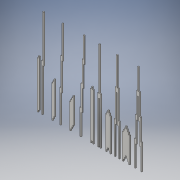
# Autodesk Inventor part: lift drawing
Saved by Autodesk Inventor 2016 SP2 (Build 200236200, 236)
## iProperties
Created: 2018-01-12
Part Number: lift drawing
Material: Generic
Document SubType Name: Modeling
Designer: CAD
Density: 1 g/cm^3
Appearance: Default
Author: CAD
Autodesk Inventor part; units mm, degrees
ref_plane "YZ Plane" through (0, 0, 0) normal (1, 0, 0) x (0, 1, 0)
ref_plane "XZ Plane" through (0, 0, 0) normal (0, 1, 0) x (-1, 0, 0)
ref_plane "XY Plane" through (0, 0, 0) normal (0, 0, 1) x (1, 0, 0)
sketch "Sketch1" plane through (0, 0, 0) normal (0, 0, 1) x (1, 0, 0)
  line L0 (0, 0) -> (2540, 0)
  line L1 (0, 0) -> (0, 1117.6)
  line L2 (0, 1117.6) -> (25.4, 1117.6)
  line L3 (25.4, 49.2125) -> (25.4, 1166.8125)
  line L4 (50.8, 49.2125) -> (50.8, 1166.8125)
  line L5 (25.4, 1166.8125) -> (50.8, 1166.8125)
  line L6 (50.8, 49.2125) -> (25.4, 49.2125)
  line L7 (25.4, 1117.6) -> (25.4, 0)
  line L8 (103.983, 0) -> (103.983, 1117.6)
  line L9 (103.983, 1117.6) -> (129.383, 1117.6)
  line L10 (129.383, 1117.6) -> (129.383, 0)
  line L11 (129.383, 1016) -> (129.383, 2133.6)
  line L12 (129.383, 2133.6) -> (154.783, 2133.6)
  line L13 (154.783, 2133.6) -> (154.783, 1016)
  line L14 (154.783, 1016) -> (129.383, 1016)
  line L15 (346.5563, 0) -> (346.5563, 774.7)
  line L16 (371.9563, 0) -> (371.9563, 774.7)
  line L17 (346.5563, 774.7) -> (371.9563, 774.7)
  line L18 (346.5563, 0) -> (371.9563, 0)
  line L19 (371.9563, 49.2125) -> (371.9563, 823.9125)
  line L20 (397.3563, 49.2125) -> (397.3563, 823.9125)
  line L21 (371.9563, 823.9125) -> (397.3563, 823.9125)
  line L22 (397.3563, 49.2125) -> (371.9563, 49.2125)
  line L23 (397.3563, 98.425) -> (397.3563, 873.125)
  line L24 (422.7563, 98.425) -> (422.7563, 873.125)
  line L25 (422.7563, 98.425) -> (397.3563, 98.425)
  line L26 (397.3563, 873.125) -> (422.7563, 873.125)
  line L27 (536.8328, 0) -> (536.8328, 774.7)
  line L28 (562.2328, 0) -> (562.2328, 774.7)
  line L29 (536.8328, 774.7) -> (562.2328, 774.7)
  line L30 (536.8328, 0) -> (562.2328, 0)
  line L31 (562.2328, 673.1) -> (562.2328, 1447.8)
  line L32 (587.6328, 673.1) -> (587.6328, 1447.8)
  line L33 (587.6328, 673.1) -> (562.2328, 673.1)
  line L34 (587.6328, 1447.8) -> (562.2328, 1447.8)
  line L35 (587.6328, 1346.2) -> (587.6328, 2120.9)
  line L36 (613.0328, 1346.2) -> (613.0328, 2120.9)
  line L37 (613.0328, 1346.2) -> (587.6328, 1346.2)
  line L38 (587.6328, 2120.9) -> (613.0328, 2120.9)
  line L39 (773.9353, 0) -> (773.9353, 609.6)
  line L40 (799.3353, 0) -> (799.3353, 609.6)
  line L41 (773.9353, 609.6) -> (799.3353, 609.6)
  line L42 (799.3353, 0) -> (773.9353, 0)
  line L43 (799.3353, 49.2125) -> (799.3353, 658.8125)
  line L44 (824.7353, 49.2125) -> (824.7353, 658.8125)
  line L45 (824.7353, 658.8125) -> (799.3353, 658.8125)
  line L46 (824.7353, 49.2125) -> (799.3353, 49.2125)
  line L47 (824.7353, 98.425) -> (824.7353, 708.025)
  line L48 (850.1353, 98.425) -> (850.1353, 708.025)
  line L49 (824.7353, 708.025) -> (850.1353, 708.025)
  line L50 (850.1353, 98.425) -> (824.7353, 98.425)
  line L51 (850.1353, 147.6375) -> (850.1353, 757.2375)
  line L52 (875.5353, 147.6375) -> (875.5353, 757.2375)
  line L53 (850.1353, 757.2375) -> (875.5353, 757.2375)
  line L54 (875.5353, 147.6375) -> (850.1353, 147.6375)
  line L55 (1020.3359, 0) -> (1020.3359, 609.6)
  line L56 (1045.7359, 0) -> (1045.7359, 609.6)
  line L57 (1045.7359, 609.6) -> (1020.3359, 609.6)
  line L58 (1020.3359, 0) -> (1045.7359, 0)
  line L59 (1045.7359, 508) -> (1045.7359, 1117.6)
  line L60 (1071.1359, 508) -> (1071.1359, 1117.6)
  line L61 (1071.1359, 508) -> (1045.7359, 508)
  line L62 (1071.1359, 1117.6) -> (1045.7359, 1117.6)
  line L63 (1071.1359, 1016) -> (1071.1359, 1625.6)
  line L64 (1096.5359, 1016) -> (1096.5359, 1625.6)
  line L65 (1096.5359, 1625.6) -> (1071.1359, 1625.6)
  line L66 (1096.5359, 1016) -> (1071.1359, 1016)
  line L67 (1096.5359, 2133.6) -> (1096.5359, 1524)
  line L68 (1121.9359, 2133.6) -> (1121.9359, 1524)
  line L69 (1096.5359, 2133.6) -> (1121.9359, 2133.6)
  line L70 (1121.9359, 1524) -> (1096.5359, 1524)
  line L71 (1631.5096, 0) -> (1631.5096, 774.7)
  line L72 (1656.9096, 0) -> (1656.9096, 774.7)
  line L73 (1631.5096, 774.7) -> (1656.9096, 774.7)
  line L74 (1631.5096, 0) -> (1656.9096, 0)
  line L75 (1656.9096, 49.2125) -> (1656.9096, 823.9125)
  line L76 (1682.3096, 49.2125) -> (1682.3096, 823.9125)
  line L77 (1656.9096, 823.9125) -> (1682.3096, 823.9125)
  line L78 (1682.3096, 49.2125) -> (1656.9096, 49.2125)
  line L79 (1682.3096, 98.425) -> (1682.3096, 873.125)
  line L80 (1707.7096, 98.425) -> (1707.7096, 873.125)
  line L81 (1707.7096, 98.425) -> (1682.3096, 98.425)
  line L82 (1682.3096, 873.125) -> (1707.7096, 873.125)
  line L83 (1733.1096, 0) -> (1733.1096, 774.7)
  line L84 (1758.5096, 0) -> (1758.5096, 774.7)
  line L85 (1733.1096, 774.7) -> (1758.5096, 774.7)
  line L86 (1733.1096, 0) -> (1758.5096, 0)
  line L87 (1733.1096, 823.9125) -> (1707.7096, 823.9125)
  line L88 (1733.1096, 49.2125) -> (1733.1096, 823.9125)
  line L89 (1707.7096, 49.2125) -> (1707.7096, 823.9125)
  line L90 (1707.7096, 49.2125) -> (1733.1096, 49.2125)
  line L91 (1836.9756, 0) -> (1836.9756, 774.7)
  line L92 (1862.3756, 0) -> (1862.3756, 774.7)
  line L93 (1836.9756, 774.7) -> (1862.3756, 774.7)
  line L94 (1836.9756, 0) -> (1862.3756, 0)
  line L95 (1862.3756, 673.1) -> (1862.3756, 1447.8)
  line L96 (1887.7756, 673.1) -> (1887.7756, 1447.8)
  line L97 (1887.7756, 673.1) -> (1862.3756, 673.1)
  line L98 (1887.7756, 1447.8) -> (1862.3756, 1447.8)
  line L99 (1887.7756, 1346.2) -> (1887.7756, 2120.9)
  line L100 (1913.1756, 1346.2) -> (1887.7756, 1346.2)
  line L101 (1887.7756, 2120.9) -> (1913.1756, 2120.9)
  line L102 (1963.9756, 0) -> (1938.5756, 0)
  line L103 (1963.9756, 0) -> (1963.9756, 774.7)
  line L104 (1938.5756, 0) -> (1938.5756, 774.7)
  line L105 (1913.1756, 1447.8) -> (1938.5756, 1447.8)
  line L106 (1963.9756, 774.7) -> (1938.5756, 774.7)
  line L107 (1938.5756, 673.1) -> (1938.5756, 1447.8)
  line L108 (1913.1756, 673.1) -> (1913.1756, 1447.8)
  line L109 (1913.1756, 673.1) -> (1938.5756, 673.1)
  line L110 (1913.1756, 2120.9) -> (1913.1756, 1346.2)
  line L111 (2031.0303, 0) -> (2031.0303, 609.6)
  line L112 (2056.4303, 0) -> (2056.4303, 609.6)
  line L113 (2031.0303, 609.6) -> (2056.4303, 609.6)
  line L114 (2056.4303, 0) -> (2031.0303, 0)
  line L115 (2056.4303, 49.2125) -> (2056.4303, 658.8125)
  line L116 (2081.8303, 49.2125) -> (2081.8303, 658.8125)
  line L117 (2081.8303, 658.8125) -> (2056.4303, 658.8125)
  line L118 (2081.8303, 49.2125) -> (2056.4303, 49.2125)
  line L119 (2081.8303, 98.425) -> (2081.8303, 708.025)
  line L120 (2107.2303, 98.425) -> (2107.2303, 708.025)
  line L121 (2081.8303, 708.025) -> (2107.2303, 708.025)
  line L122 (2107.2303, 98.425) -> (2081.8303, 98.425)
  line L123 (2107.2303, 147.6375) -> (2107.2303, 757.2375)
  line L124 (2107.2303, 757.2375) -> (2132.6303, 757.2375)
  line L125 (2132.6303, 147.6375) -> (2107.2303, 147.6375)
  line L126 (2158.0303, 49.2125) -> (2183.4303, 49.2125)
  line L127 (2132.6303, 98.425) -> (2158.0303, 98.425)
  line L128 (2158.0303, 98.425) -> (2158.0303, 708.025)
  line L129 (2132.6303, 98.425) -> (2132.6303, 708.025)
  line L130 (2208.8303, 0) -> (2208.8303, 609.6)
  line L131 (2183.4303, 0) -> (2208.8303, 0)
  line L132 (2183.4303, 49.2125) -> (2183.4303, 658.8125)
  line L133 (2183.4303, 0) -> (2183.4303, 609.6)
  line L134 (2158.0303, 49.2125) -> (2158.0303, 658.8125)
  line L135 (2208.8303, 609.6) -> (2183.4303, 609.6)
  line L136 (2158.0303, 658.8125) -> (2183.4303, 658.8125)
  line L137 (2158.0303, 708.025) -> (2132.6303, 708.025)
  line L138 (2132.6303, 757.2375) -> (2132.6303, 147.6375)
  line L139 (2319.4925, 0) -> (2319.4925, 609.6)
  line L140 (2344.8925, 0) -> (2344.8925, 609.6)
  line L141 (2344.8925, 609.6) -> (2319.4925, 609.6)
  line L142 (2319.4925, 0) -> (2344.8925, 0)
  line L143 (2344.8925, 508) -> (2344.8925, 1117.6)
  line L144 (2370.2925, 508) -> (2370.2925, 1117.6)
  line L145 (2370.2925, 508) -> (2344.8925, 508)
  line L146 (2370.2925, 1117.6) -> (2344.8925, 1117.6)
  line L147 (2370.2925, 1016) -> (2370.2925, 1625.6)
  line L148 (2395.6925, 1016) -> (2395.6925, 1625.6)
  line L149 (2395.6925, 1625.6) -> (2370.2925, 1625.6)
  line L150 (2395.6925, 1016) -> (2370.2925, 1016)
  line L151 (2395.6925, 2133.6) -> (2395.6925, 1524)
  line L152 (2395.6925, 2133.6) -> (2421.0925, 2133.6)
  line L153 (2421.0925, 1524) -> (2395.6925, 1524)
  line L154 (2471.8925, 609.6) -> (2497.2925, 609.6)
  line L155 (2471.8925, 0) -> (2471.8925, 609.6)
  line L156 (2497.2925, 0) -> (2497.2925, 609.6)
  line L157 (2497.2925, 0) -> (2471.8925, 0)
  line L158 (2421.0925, 1625.6) -> (2446.4925, 1625.6)
  line L159 (2421.0925, 1016) -> (2446.4925, 1016)
  line L160 (2421.0925, 1016) -> (2421.0925, 1625.6)
  line L161 (2446.4925, 1117.6) -> (2471.8925, 1117.6)
  line L162 (2446.4925, 1016) -> (2446.4925, 1625.6)
  line L163 (2471.8925, 508) -> (2471.8925, 1117.6)
  line L164 (2446.4925, 508) -> (2446.4925, 1117.6)
  line L165 (2446.4925, 508) -> (2471.8925, 508)
  line L166 (2421.0925, 2133.6) -> (2421.0925, 1524)
  line L167 (1270, 0) -> (1270, 1117.6)
  line L168 (1270, 1117.6) -> (1295.4, 1117.6)
  line L169 (1295.4, 49.2125) -> (1295.4, 1166.8125)
  line L170 (1295.4, 1166.8125) -> (1320.8, 1166.8125)
  line L171 (1320.8, 49.2125) -> (1295.4, 49.2125)
  line L172 (1295.4, 1117.6) -> (1295.4, 0)
  line L173 (1320.8, 1117.6) -> (1320.8, 0)
  line L174 (1346.2, 0) -> (1346.2, 1117.6)
  line L175 (1346.2, 1117.6) -> (1320.8, 1117.6)
  line L176 (1320.8, 1166.8125) -> (1320.8, 49.2125)
  line L177 (1320.8, 0) -> (1346.2, 0)
  line L178 (1270, 0) -> (1295.4, 0)
  line L179 (1346.2, 1117.6) -> (1320.8, 1117.6)
  line L180 (1295.4, 1117.6) -> (1270, 1117.6)
  line L181 (1442.8758, 0) -> (1442.8758, 1117.6)
  line L182 (1442.8758, 1117.6) -> (1468.2758, 1117.6)
  line L183 (1468.2758, 1016) -> (1468.2758, 0)
  line L184 (1468.2758, 1117.6) -> (1468.2758, 2133.6)
  line L185 (1468.2758, 2133.6) -> (1493.6758, 2133.6)
  line L186 (1493.6758, 1016) -> (1468.2758, 1016)
  line L187 (1519.0758, 1117.6) -> (1519.0758, 0)
  line L188 (1493.6758, 1117.6) -> (1519.0758, 1117.6)
  line L189 (1493.6758, 2133.6) -> (1493.6758, 1117.6)
  line L190 (1493.6758, 1016) -> (1493.6758, 0)
  line L191 (1468.2758, 1117.6) -> (1468.2758, 1016)
  line L192 (1493.6758, 1016) -> (1493.6758, 1117.6)
  line L193 (1442.8758, 0) -> (1468.2758, 0)
  line L194 (1493.6758, 0) -> (1519.0758, 0)
  dimension "d0" = 2540
  dimension "d1" = 1117.6
  dimension "d4" = 1117.6
  dimension "d5" = 25.4
  dimension "d6" = 0
  dimension "d7" = 49.2125
  dimension "d8" = 25.4
  dimension "d9" = 25.4
  dimension "d11" = 101.6
  dimension "d12" = 25.4
  dimension "d13" = 1117.6
  dimension "d14" = 1117.6
  dimension "d15" = 103.983
  dimension "d18" = 25.4
  dimension "d19" = 346.5563
  dimension "d21" = 774.7
  dimension "d22" = 49.2125
  dimension "d23" = 25.4
  dimension "d24" = 774.7
  dimension "d25" = 25.4
  dimension "d26" = 49.2125
  dimension "d27" = 49.2125
  dimension "d29" = 25.4
  dimension "d30" = 536.8328
  dimension "d31" = 774.7
  dimension "d32" = 25.4
  dimension "d33" = 101.6
  dimension "d34" = 774.7
  dimension "d35" = 25.4
  dimension "d36" = 25.4
  dimension "d39" = 25.4
  dimension "d41" = 49.2125
  dimension "d42" = 25.4
  dimension "d43" = 0
  dimension "d44" = 609.6
  dimension "d45" = 25.4
  dimension "d46" = 609.6
  dimension "d47" = 49.2125
  dimension "d48" = 25.4
  dimension "d49" = 609.6
  dimension "d50" = 25.4
  dimension "d51" = 609.6
  dimension "d52" = 101.6
  dimension "d53" = 25.4
  dimension "d54" = 221.0006
  dimension "d55" = 773.9353
  dimension "d56" = 609.6
  dimension "d57" = 101.6
  dimension "d58" = 25.4
  dimension "d60" = 101.6
  dimension "d61" = 25.4
  dimension "d64" = 101.6
  dimension "d95" = 49.2125
  dimension "d99" = 49.2125
  dimension "d100" = 49.2125
  dimension "d113" = 0
  dimension "d114" = 0
  dimension "d115" = 25.4
  dimension "d116" = 774.7
  dimension "d117" = 25.4
  dimension "d118" = 101.6
  dimension "d119" = 774.7
  dimension "d120" = 25.4
  dimension "d122" = 101.6
  constraints: 388 end point, 80 parallel, 35 vertical, 31 horizontal, 18 point on line, 11 collinear, 10 perpendicular, 12 other
  measures "d0" distance of point (0, 0) point (2540, 0)
  measures "d1" distance of L1.start L1.end
  measures "d4" distance of L3.start L3.end
  measures "d5" distance between parallel lines of L3 L4
  measures "d6" distance of point (0, 0) L1.start
  measures "d7" vertical distance of point (0, 0) L3.start
  measures "d8" distance of L1.end L2.end
  measures "d9" distance of L8.end L9.end
  measures "d11" vertical distance of L8.end L11.start
  measures "d12" distance of L11.end L12.end
  measures "d13" distance of L12.end L13.end
  measures "d14" distance of L8.start L8.end
  measures "d15" distance from line of point (0, 0) L8
  measures "d18" distance between parallel lines of L15 L16
  measures "d19" distance of point (0, 0) L15.start
  measures "d21" distance of L19.start L19.end
  measures "d22" distance of L16.start L19.start
  measures "d23" distance between parallel lines of L19 L20
  measures "d24" distance of L23.start L23.end
  measures "d25" distance between parallel lines of L23 L24
  measures "d26" vertical distance of L20.start L24.start
  measures "d27" distance of L20.end L23.end
  measures "d29" distance between parallel lines of L27 L28
  measures "d30" distance of point (0, 0) L27.start
  measures "d31" distance of L31.start L31.end
  measures "d32" distance between parallel lines of L31 L32
  measures "d33" vertical distance of L27.end L31.start
  measures "d34" distance of L35.start L35.end
  measures "d35" distance from line of L31.end L35
  measures "d36" distance between parallel lines of L35 L36
  measures "d39" distance between parallel lines of L39 L40
  measures "d41" distance of L40.start L43.start
  measures "d42" distance between parallel lines of L43 L44
  measures "d43" distance between parallel lines of L44 L47
  measures "d44" distance of L47.start L47.end
  measures "d45" distance between parallel lines of L47 L48
  measures "d46" distance of L51.start L51.end
  measures "d47" distance of L48.start L51.start
  measures "d48" distance between parallel lines of L51 L52
  measures "d49" distance of L55.start L55.end
  measures "d50" distance between parallel lines of L55 L56
  measures "d51" distance of L59.start L59.end
  measures "d52" vertical distance of L55.end L59.start
  measures "d53" distance between parallel lines of L59 L60
  measures "d54" distance of L40.start L55.start
  measures "d55" distance of point (0, 0) L39.start
  measures "d56" distance of L63.start L63.end
  measures "d57" vertical distance of L59.end L63.start
  measures "d58" distance between parallel lines of L63 L64
  measures "d60" vertical distance of L63.end L67.end
  measures "d61" distance between parallel lines of L67 L68
  measures "d64" vertical distance of L31.end L35.start
  measures "d95" distance of L72.start L75.start
  measures "d99" vertical distance of L76.start L80.start
  measures "d100" distance of L77.end L79.end
  measures "d113" distance between parallel lines of L80 L89
  measures "d114" distance between parallel lines of L88 L83
  measures "d115" distance between parallel lines of L91 L92
  measures "d116" distance of L95.start L98.end
  measures "d117" distance between parallel lines of L95 L96
  measures "d118" vertical distance of L91.end L95.start
  measures "d119" distance of L100.end L99.end
  measures "d120" distance from line of L98.end L99
  measures "d122" vertical distance of L98.end L100.end
extrude "Extrusion1" add sketch "Sketch1" along normal blind 25.4 contours L1 L2 L3 L7 L0 | L139 L141 L140 L0 | L111 L113 L112 L0 | L91 L93 L92 L0 | L71 L73 L72 L0 | L181 L182 L191 L183 L0 | L167 L168 L169 L172 L0 | L55 L57 L56 L0 | L39 L41 L40 L0 | L27 L29 L28 L0 | L15 L17 L16 L0 | L8 L9 L10 L0 | L3 L5 L4 L6 | L10 L11 L12 L13 L14 | L16 L19 L21 L20 L22 | L28 L31 L34 L32 L33 | L20 L23 L26 L24 L25 | L40 L43 L45 L44 L46 | L32 L35 L38 L36 L37 | L56 L59 L62 L60 L61 | L44 L47 L49 L48 L50 | L173 L175 L174 L0 | L169 L170 L176 L173 L171 | L60 L63 L65 L64 L66 | L48 L51 L53 L52 L54 | L64 L67 L69 L68 L70 | L190 L192 L188 L187 L0 | L191 L184 L185 L189 L192 L186 | L83 L85 L84 L0 | L72 L75 L77 L76 L78 | L90 L89 L80 L87 L88 L83 | L76 L79 L82 L80 L81 | L104 L106 L103 L0 | L92 L95 L98 L96 L97 | L109 L108 L105 L107 L104 | L96 L99 L101 L110 L108 L100 | L133 L132 L135 L130 L0 | L112 L115 L117 L116 L118 | L126 L134 L128 L136 L132 | L116 L119 L121 L120 L122 | L127 L129 L137 L128 | L155 L154 L156 L0 | L140 L143 L146 L144 L145 | L120 L123 L124 L138 L129 L125 | L165 L164 L162 L161 L163 L155 | L144 L147 L149 L148 L150 | L159 L160 L158 L162 | L148 L151 L152 L166 L160 L153
equation "\"d21\" = d17"
equation "\"d22\" = d7"
equation "\"d24\" = d17"
equation "\"d26\" = d22"
equation "\"d31\" = d17"
equation "\"d34\" = d17"
equation "\"d41\" = d26"
equation "\"d44\" = d40"
equation "\"d46\" = d44"
equation "\"d47\" = d41"
equation "\"d49\" = d46"
equation "\"d51\" = d46"
equation "\"d56\" = d46"
equation "\"d57\" = d52"
equation "\"d60\" = d57"
equation "\"d95\" = d102"
equation "\"d99\" = d95"
equation "\"d40\" = d38"
equation "\"d17\" = 774.7"
equation "\"d102\" = 49.2125"
equation "\"d38\" = 609.6"
body "Solid1"
